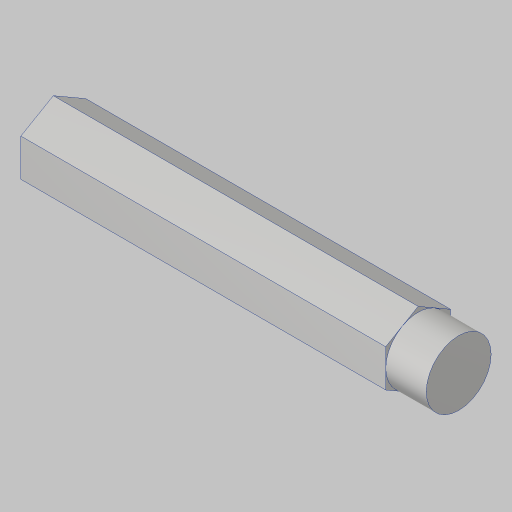
# Autodesk Inventor part: EL2-CGB-004
Saved by Autodesk Inventor 2023.5 (Build 275446000, 446)
## iProperties
Created: 2025-01-19
Part Number: EL2-CGB-004
Material: Aluminum 6061
Document SubType Name: Modeling
Designer: mavericks
Density: 2.7 g/cm^3
Appearance: Aluminum - Flat
Author: mavericks
Autodesk Inventor part; units mm, degrees
ref_plane "YZ Plane" through (0, 0, 0) normal (1, 0, 0) x (0, 1, 0)
ref_plane "XZ Plane" through (0, 0, 0) normal (0, 1, 0) x (-1, 0, 0)
ref_plane "XY Plane" through (0, 0, 0) normal (0, 0, 1) x (1, 0, 0)
sketch "Sketch1" plane through (0, 0, 0) normal (1, 0, 0) x (0, 1, 0)
  line L0 (3.6662, 6.35) -> (7.3323, 0)
  line L1 (7.3323, 0) -> (3.6662, -6.35)
  line L2 (3.6662, -6.35) -> (-3.6662, -6.35)
  line L3 (-3.6662, -6.35) -> (-7.3323, 0)
  line L4 (-7.3323, 0) -> (-3.6662, 6.35)
  line L5 (-3.6662, 6.35) -> (3.6662, 6.35)
  point P0 (0, 0)
  point P1 (0, 0)
  dimension "d0" = 12.7
  constraints: 12 end point, 1 coincident, 1 horizontal, 13 other
  measures "d0" distance between parallel lines of L2 L5
extrude "Extrusion1" add sketch "Sketch1" along normal mid plane 79.375
sketch "Sketch2" plane through (39.6875, 0, 0) normal (1, 0, 0) x (0, 0, -1)
  line L0 (-6.35, -3.6662) -> (0, -7.3323) projected
  line L1 (0, -7.3323) -> (6.35, -3.6662) projected
  line L2 (6.35, -3.6662) -> (6.35, 3.6662) projected
  line L3 (6.35, 3.6662) -> (0, 7.3323) projected
  line L4 (0, 7.3323) -> (-6.35, 3.6662) projected
  line L5 (-6.35, 3.6662) -> (-6.35, -3.6662) projected
  circle A0 centre (0, 0) radius 6.35
  point P0 (-3.175, 5.4993)
  point P1 (3.175, 5.4993)
  point P2 (6.35, 0)
  point P3 (3.175, -5.4993)
  point P4 (-3.175, -5.4993)
  point P5 (-6.35, 0)
  dimension "d3" = 12.7
  constraints: 1 centre point, 1 coincident
  measures "d3" diameter of A0
extrude "Extrusion2" cut sketch "Sketch2" against normal blind 7.9375 contours L5 A0 L0 | A0 L1 L0 | L5 L4 A0 | A0 L2 L1 | L4 L3 A0 | A0 L3 L2
body "Solid1"
